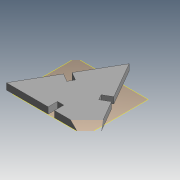
# Autodesk Inventor part: Lower PlatformV
Saved by Autodesk Inventor 2014 SP1 (Build 180222100, 222)
## iProperties
Created: 2014-04-09
Part Number: Lower PlatformV
Material: Generic
Document SubType Name: Modeling
Designer: tom
Density: 1 g/cm^3
Appearance: Default
Author: tom
Autodesk Inventor part; units mm, degrees
ref_plane "YZ Plane" through (0, 0, 0) normal (1, 0, 0) x (0, 1, 0)
ref_plane "XZ Plane" through (0, 0, 0) normal (0, 1, 0) x (-1, 0, 0)
ref_plane "XY Plane" through (0, 0, 0) normal (0, 0, 1) x (1, 0, 0)
ref_plane "Work Plane1" through (64.8465, 16.6938, -6.1656) normal (0, 1, 0) x (1, 0, 0)
sketch "Sketch1" plane through (64.8465, 16.6938, -6.1656) normal (0, 1, 0) x (1, 0, 0)
  line L0 (1.7321, 1) -> (27.6872, 15.9852) construction
  line L1 (13.1559, 10.8634) -> (20.3785, 15.0334)
  line L2 (15.9859, 5.9616) -> (23.2085, 10.1316)
  line L3 (13.1559, 10.8634) -> (15.9859, 5.9616)
  circle A0 centre (1.7321, 1) radius 20 construction
  circle A1 centre (19.0526, 11) radius 5.175 construction
  circle A2 centre (1.7321, 1) radius 1.5
  line L4 (1.7321, 1) -> (8.6603, 5) construction
  circle A3 centre (8.6603, 5) radius 1.5
  line L5 (17.3785, 20.2295) -> (1.7321, 11.196)
  line L6 (1.7321, 11.196) -> (-13.9144, 20.2295)
  line L7 (26.2085, 4.9355) -> (10.5621, -4.098)
  circle A4 centre (1.7321, 1) radius 10.196 construction
  line L8 (-12.5218, 5.9616) -> (-19.7444, 10.1316)
  line L9 (-9.6918, 10.8634) -> (-16.9144, 15.0334)
  line L10 (-12.5218, 5.9616) -> (-9.6918, 10.8634)
  circle A5 centre (-5.1962, 5) radius 1.5
  line L11 (4.5621, -13.825) -> (4.5621, -22.165)
  line L12 (-1.0979, -13.825) -> (-1.0979, -22.165)
  line L13 (4.5621, -13.825) -> (-1.0979, -13.825)
  circle A6 centre (1.7321, -7) radius 1.5
  line L14 (-7.0979, -22.165) -> (-7.0979, -4.098)
  line L15 (10.5621, -22.165) -> (10.5621, -4.098)
  line L16 (-7.0979, -4.098) -> (-22.7444, 4.9355)
  line L17 (-7.0979, -22.165) -> (-1.0979, -22.165)
  line L18 (4.5621, -22.165) -> (10.5621, -22.165)
  line L19 (-13.9144, 20.2295) -> (-16.9144, 15.0334)
  line L20 (-19.7444, 10.1316) -> (-22.7444, 4.9355)
  line L21 (17.3785, 20.2295) -> (20.3785, 15.0334)
  line L22 (23.2085, 10.1316) -> (26.2085, 4.9355)
  dimension "d34" = 40
  dimension "d35" = 10.35
  dimension "d45" = 3
  dimension "d47" = 8
  dimension "d48" = 3
  dimension "d54" = 360
  constraints: 46 end point, 6 centre point, 6 perpendicular, 4 coincident, 3 point on circle, 2 parallel, 2 point on line, 31 other
  measures "d35" diameter of A1
  measures "d45" diameter of A2
  measures "d47" distance of L4.start L4.end
  measures "d48" diameter of A3
extrude "Extrusion2" add sketch "Sketch1" along normal blind 5.66
fillet "Fillet1" radius 3 3 edges at (75.4086, 19.5238, -2.0676) (66.5786, 19.5238, -17.3616) (57.7486, 19.5238, -2.0676)
fillet "Fillet2" radius 3 2 edges at (91.055, 19.5238, -11.1011) (82.225, 19.5238, -26.3951)
pattern_circular "Circular Pattern1" count 3 over 360 about axis through (66.5786, 16.6938, -7.1656) along (0, 1, 0) of "Fillet2"
body "Solid2"
